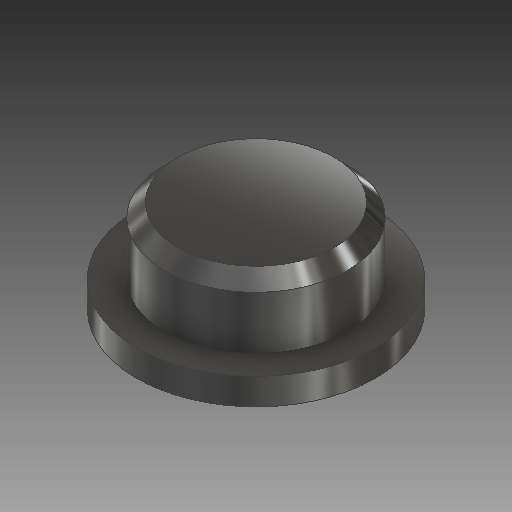
# Autodesk Inventor part: Servorückseitenlagerachse
Saved by Autodesk Inventor 2018 (Build 220112000, 112)
## iProperties
Part Number: Servorückseitenlagerachse
Material: Siliziumnitrid
Document SubType Name: Modeling
Designer: Jochen Alt
Mass: 0.491375 g
Surface Area: 2.03027 cm^2
Volume: 0.154521 cm^3
Density: 3.18 g/cm^3
Appearance: Chrom - poliert - schwarz
Author: Jochen Alt
Autodesk Inventor part; units mm, degrees
ref_plane "YZ Plane" through (0, 0, 0) normal (1, 0, 0) x (0, 1, 0)
ref_plane "XZ Plane" through (0, 0, 0) normal (0, 1, 0) x (-1, 0, 0)
ref_plane "XY Plane" through (0, 0, 0) normal (0, 0, 1) x (1, 0, 0)
sketch "Skizze1" plane through (0, 0, 0) normal (0, 0, 1) x (1, 0, 0)
  circle A0 centre (0, 0) radius 4.5
  dimension "d0" = 9
  constraints: 1 centre point, 1 coincident
  measures "d0" diameter of A0
extrude "Extrusion1" add sketch "Skizze1" along normal blind 1
sketch "Skizze2" plane through (0, 0, 1) normal (0, 0, 1) x (1, 0, 0)
  circle A0 centre (0, 0) radius 4.5 projected
  circle A1 centre (0, 0) radius 3.45
  dimension "d3" = 6.9
  constraints: 1 centre point, 1 coincident
  measures "d3" diameter of A1
extrude "Extrusion2" add sketch "Skizze2" along normal blind 2.5 contours A1
chamfer "Fase2" distance 0.5 angle 45 1 edges at (-3.45, 0, 3.5)
